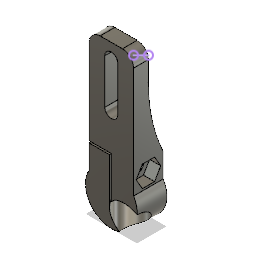
EndoHalter (Autodesk Fusion 360 design; units mm, degrees)
Autodesk Fusion 360 part; units mm, degrees
sketch "Skizze1" plane through (0, 0, 0) normal (0, 0, 1) x (1, 0, 0)
  line L0 (6, 20) -> (-6, 20)
  line L1 (-6, 20) -> (-6, -20)
  line L2 (-6, -20) -> (6, -20)
  line L3 (6, -20) -> (6, 20)
  line L4 (6, 20) -> (-6, -20) construction
  line L5 (-6, 20) -> (6, -20) construction
  dimension "d1" = 12
  dimension "d2" = 40
  constraint horizontal L0
  constraint perpendicular L0 L1
  constraint parallel L0 L2
  constraint parallel L1 L3
  constraint coincident L4 origin
  constraint coincident L5 origin
  measures "d1" distance of L1.end L2.end
  measures "d2" distance of L0.end L1.end
extrude "Extrusion1" add sketch "Skizze1" along normal blind 4
sketch "Skizze2" plane through (0, 0, 4) normal (0, 0, 1) x (1, 0, 0)
  line L0 (6, -20) -> (6, 20)
  line L1 (6, 20) -> (-6, 20)
  line L2 (-6, 20) -> (-6, -20)
  line L3 (-6, -20) -> (6, -20)
  circle A0 centre (0, -16.3944) radius 7
  dimension "d5" = 6
  dimension "d6" = 14
  constraint coincident L2.end A0
  measures "d5" distance of L2 A0.centre
  measures "d6" diameter of A0
extrude "Extrusion2" add sketch "Skizze2" against normal up to surface (4 mm away) contours L3 A0 | L0 A0 | L2 A0
sketch "Skizze3" plane through (0, 0, 0) normal (0, 0, -1) x (-1, 0, 0)
  arc A0 (-6, -12.7889) -> (6, -12.7889) centre (0, -16.3944) ccw
  line L0 (6, -12.7889) -> (6, 20)
  line L1 (6, 20) -> (-6, 20)
  line L2 (-6, 20) -> (-6, -12.7889)
  line L3 (-6, -6.3944) -> (6, -6.3944)
  dimension "d9" = 10
  constraint coincident L2 L3.start
  constraint coincident L0 L3.end
  constraint perpendicular L0 L3
  measures "d9" distance of A0.centre L3
extrude "Extrusion3" add sketch "Skizze3" along normal blind 4 contours A0 L0 L2 L3
ref_plane "Arbeitsebene1" through (6, 3.6056, 4) normal (0.707107, 0, 0.707107) x (0, 1, 0)
sketch "Skizze4" plane through (6, 3.6056, 4) normal (0.707107, 0, 0.707107) x (0, 1, 0)
  line L0 (16.3944, -2.8284) -> (16.3944, 0)
ref_plane "Arbeitsebene2" through (7, 20, 3) normal (0.664463, -0.34202, 0.664463) x (-0.707107, 0, 0.707107)
sketch "Skizze5" plane through (7, 20, 3) normal (0.664463, -0.34202, 0.664463) x (-0.707107, 0, 0.707107)
  circle A0 centre (2, 38) radius 4
  dimension "d14" = 8
  dimension "d15" = 2
  dimension "d16" = 38
  measures "d14" diameter of A0
  measures "d15" horizontal distance of origin A0.centre
  measures "d16" vertical distance of origin A0.centre
extrude "Extrusion4" cut sketch "Skizze5" along normal mid plane 70
sketch "Skizze6" plane through (0, 0, -4) normal (0, 0, -1) x (-1, 0, 0)
  ellipse E0 centre (2.8284, -16.1077) end of major axis (8.1809, -13.3526) minor radius 4 (6, -11.7667) -> (6.7796, -18.137) ccw
  line L0 (6, -6.3944) -> (-6, -6.3944)
  line L1 (-6, -6.3944) -> (-6, -12.7889)
  arc A0 (-6, -12.7889) -> (6.7796, -18.137) centre (0, -16.3944) ccw
  line L2 (6, -6.3944) -> (0, -6.3944)
  line L3 (0, -6.3944) -> (0, -5.8944)
  line L4 (0, -5.8944) -> (6, -5.8944)
  line L5 (6, -5.8944) -> (6, -6.3944)
  line L6 (0, -6.3944) -> (0.5, -6.3944)
  line L7 (0.5, -6.3944) -> (0.5, -18.3944)
  line L8 (0.5, -18.3944) -> (0, -18.3944)
  line L9 (0, -18.3944) -> (0, -6.3944)
  line L10 (6, -11.7667) -> (6, -6.3944)
  dimension "d19" = 0.5
  dimension "d20" = 0.5
  dimension "d21" = 12
  constraint horizontal L2
  constraint vertical L3
  constraint horizontal L4
  constraint vertical L5
  constraint coincident L0.start L2.start
  constraint coincident origin L3
  constraint horizontal L6
  constraint vertical L7
  constraint horizontal L8
  constraint vertical L9
  measures "d19" distance of L0.start L4.end
  measures "d20" distance of L2.end L6.end
  measures "d21" distance of L2.end L8.end
extrude "Extrusion5" cut sketch "Skizze6" against normal blind 9 contours E0 L7 L8 L9 | E0 L0 L2 L6 L7 L9 | L0 L2 L3 L4 L5 L6
sketch "Skizze7" plane through (-6, 0, 0) normal (-1, 0, 0) x (0, 0, 1)
  line L0 (4, -6.3944) -> (-4, -6.3944)
  line L1 (-2.8955, -12.7889) -> (4, -12.7889)
  line L2 (4, -12.7889) -> (4, -6.3944)
  circle A0 centre (0, -9.3944) radius 1.7
  ellipse E0 centre (-7.1716, -14.4752) end of major axis (-1.8191, -17.2303) minor radius 4 (-2.8955, -12.7889) -> (-4, -11.7667) ccw
  line L3 (-4, -6.3944) -> (-4, -11.7667)
  dimension "d24" = 3.4
  dimension "d25" = 4
  dimension "d26" = 3
  measures "d24" diameter of A0
  measures "d25" distance of L2 A0.centre
  measures "d26" distance of L0 A0.centre
extrude "Extrusion6" cut sketch "Skizze7" against normal blind 18 contours A0
sketch "Skizze8" plane through (6, 0, 0) normal (1, 0, 0) x (0, 0, -1)
  circle A0 centre (0, -9.3944) radius 1.7
  line L0 (-4, -12.7889) -> (4, -12.7889)
  line L1 (4, -12.7889) -> (4, -6.3944)
  line L2 (4, -6.3944) -> (0, -6.3944)
  line L3 (0, -6.3944) -> (0, 20)
  line L4 (0, 20) -> (-4, 20)
  line L5 (-4, 20) -> (-4, -12.7889)
  line L6 (1.6454, -6.5444) -> (-1.6454, -6.5444)
  line L7 (-1.6454, -6.5444) -> (-3.2909, -9.3944)
  line L8 (-3.2909, -9.3944) -> (-1.6454, -12.2444)
  line L9 (-1.6454, -12.2444) -> (1.6454, -12.2444)
  line L10 (1.6454, -12.2444) -> (3.2909, -9.3944)
  line L11 (3.2909, -9.3944) -> (1.6454, -6.5444)
  point P0 (0, -9.3944)
  dimension "d29" = 5.7
  constraint coincident P0 A0.centre
  constraint horizontal L6
  measures "d29" distance of L7 L10
extrude "Extrusion7" cut sketch "Skizze8" against normal blind 3 contours L6 L7 L8 L9 L10 L11
fillet "Abrundung1" radius 43 1 edges at (3, -6.3944, 0)
sketch "Skizze9" plane through (0, 0, 0) normal (0, 0, -1) x (-1, 0, 0)
  line L0 (-6, 11.7163) -> (6, 11.7163)
  line L1 (6, 11.7163) -> (6, 20)
  line L2 (6, 20) -> (-6, 20)
  line L3 (-6, 20) -> (-6, 11.7163)
  line L4 (-1.75, 16) -> (-1.75, 4)
  arc A0 (-1.75, 4) -> (1.75, 4) centre (0, 4) ccw
  line L5 (1.75, 4) -> (1.75, 16)
  arc A1 (1.75, 16) -> (-1.75, 16) centre (0, 16) ccw
  line L6 (0, 16) -> (0, 4) construction
  dimension "d34" = 3.5
  dimension "d35" = 12
  dimension "d36" = 4
  constraint tangent L4 A0
  constraint tangent A0 L5
  constraint parallel L4 L5
  constraint tangent L5 A1
  constraint tangent L4 A1
  constraint perpendicular L0 L6
  measures "d34" diameter of A0
  measures "d35" distance of A0.end L5.end
  measures "d36" distance of L2 A1.centre
extrude "Extrusion8" cut sketch "Skizze9" along normal mid plane 20 contours L0 L4 L5 A1 | L0 L4 A0 L5
sketch "Skizze10" plane through (0, 0, 0) normal (0, 0, -1) x (-1, 0, 0)
  line L0 (-1.75, 11.7163) -> (-1.75, 16)
  arc A0 (1.75, 16) -> (-1.75, 16) centre (0, 16) ccw
  line L1 (1.75, 16) -> (1.75, 11.7163)
  line L2 (1.75, 11.7163) -> (6, 11.7163)
  line L3 (6, 11.7163) -> (6, 20)
  line L4 (6, 20) -> (-6, 20)
  line L5 (-6, 20) -> (-6, 11.7163)
  line L6 (-6, 11.7163) -> (-1.75, 11.7163)
  line L7 (-3.5, 16) -> (-3.5, 4)
  arc A1 (-3.5, 4) -> (3.5, 4) centre (0, 4) ccw
  line L8 (3.5, 4) -> (3.5, 16)
  arc A2 (3.5, 16) -> (-3.5, 16) centre (0, 16) ccw
  line L9 (0, 16) -> (0, 4) construction
  dimension "d39" = 3.5
  constraint tangent L7 A1
  constraint tangent A1 L8
  constraint parallel L7 L8
  constraint tangent L8 A2
  constraint tangent L7 A2
  constraint perpendicular L4 L9
  constraint coincident A0.centre A2.centre
  measures "d39" radius of A2
extrude "Extrusion9" cut sketch "Skizze10" along normal blind 5 contours L0 A0 L1 L2 L6 L7 A1 L8
fillet "Abrundung2" radius 3 2 edges at (-6, 20, 2) (6, 20, 2)
